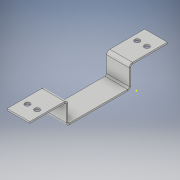
# Autodesk Inventor part: Hew battery holder
Saved by Autodesk Inventor 2017 (Build 210142000, 142)
## iProperties
Created: 2016-10-03
Part Number: Hew battery holder
Material: Generic
Document SubType Name: Sheet Metal
Designer: situh
Density: 1 g/cm^3
Sheet Metal Rule: Default
Appearance: Default
Author: situh
Autodesk Inventor part; units mm, degrees
ref_plane "YZ Plane" through (0, 0, 0) normal (1, 0, 0) x (0, 1, 0)
ref_plane "XZ Plane" through (0, 0, 0) normal (0, 1, 0) x (-1, 0, 0)
ref_plane "XY Plane" through (0, 0, 0) normal (0, 0, 1) x (1, 0, 0)
sketch "Sketch1" plane through (0, 0, 0) normal (0, 0, 1) x (1, 0, 0)
  line L0 (-22.189, 41.743) -> (-4.409, 41.743)
  line L1 (-4.409, 41.743) -> (-4.409, 23.963)
  line L2 (-4.409, 23.963) -> (-22.189, 23.963)
  line L3 (-22.189, 23.963) -> (-22.189, 41.743)
  point P0 (0, 0)
  dimension "d0" = 17.78
  dimension "d1" = 17.78
  measures "d0" distance of L2.end L0.start
  measures "d1" distance of L0.start L0.end
extrude "Plate1" add sketch "Sketch1" along normal blind 1.27
sketch "Sketch2" plane through (-4.409, 40.473, 1.27) normal (0, 1, 0) x (-1, 0, 0)
  line L0 (17.78, 0) -> (0, 0)
  line L1 (0, 0) -> (0, -30)
  line L2 (0, -30) -> (17.78, -30)
  line L3 (17.78, -30) -> (17.78, 0)
  constraints: 6 end point, 1 horizontal, 1 perpendicular, 1 vertical
edge flange "Flange1" height 30 angle 90 thickness 1.27 bend radius 1.27 thickness toward (0, 1, 0) relief straight relief width 1.27 relief depth 0.635 edges at (-13.299, 41.743, 0) wall of the first edge with corners at (-22.189, 40.473, 1.27) (-4.409, 40.473, 1.27) (-4.409, 40.473, -28.73) (-22.189, 40.473, -28.73)
bend "Bend1"
corner "Corner1"
sketch "Sketch4" plane through (-22.189, 41.743, -28.73) normal (0, 1, 0) x (1, 0, 0)
  circle A0 centre (12.7, -10.95) radius 2
  circle A1 centre (5.08, -10.95) radius 2
  line L0 (17.78, 0) -> (17.78, -27.46) projected
  line L1 (0, -27.46) -> (0, 0) projected
  line L2 (0, -27.46) -> (17.78, -27.46) projected
  point P0 (22.189, -28.73)
  dimension "d26" = 4
  dimension "d27" = 4
  dimension "d29" = 5.08
  dimension "d30" = 5.08
  dimension "d31" = 16.51
  dimension "d32" = 16.51
  constraints: 2 centre point
  measures "d26" diameter of A1
  measures "d27" diameter of A0
  measures "d29" distance from line of A0.centre L0
  measures "d30" distance from line of L1 A1.centre
  measures "d31" distance from line of L2 A1.centre
  measures "d32" vertical distance of L0.end A0.centre
extrude "Extrusion2" cut sketch "Sketch4" against normal blind 2.54
sketch "Sketch5" plane through (-4.409, 25.233, 0) normal (0, -1, 0) x (1, 0, 0)
  line L0 (-17.78, 0) -> (0, 0)
  line L1 (0, 0) -> (0, 50.8)
  line L2 (0, 50.8) -> (-17.78, 50.8)
  line L3 (-17.78, 50.8) -> (-17.78, 0)
  constraints: 6 end point, 1 horizontal, 1 perpendicular, 1 vertical
edge flange "Flange2" height 50.8 angle 90 thickness 1.27 bend radius 1.27 thickness toward (0, -1, 0) relief straight relief width 1.27 relief depth 0.635 edges at (-13.299, 23.963, 1.27) wall of the first edge with corners at (-22.189, 25.233, 0) (-4.409, 25.233, 0) (-4.409, 25.233, 50.8) (-22.189, 25.233, 50.8)
bend "Bend2"
corner "Corner2"
sketch "Sketch6" plane through (-4.409, 23.963, 49.53) normal (0, 0, 1) x (1, 0, 0)
  line L0 (-17.78, 0) -> (0, 0)
  line L1 (0, 0) -> (0, 15.24)
  line L2 (0, 15.24) -> (-17.78, 15.24)
  line L3 (-17.78, 15.24) -> (-17.78, 0)
  constraints: 6 end point, 1 horizontal, 1 perpendicular, 1 vertical
edge flange "Flange3" height 15.24 angle 90 thickness 1.27 bend radius 1.27 thickness toward (0, 0, 1) relief straight relief width 1.27 relief depth 0.635 edges at (-13.299, 25.233, 50.8) wall of the first edge with corners at (-22.189, 23.963, 49.53) (-4.409, 23.963, 49.53) (-4.409, 39.203, 49.53) (-22.189, 39.203, 49.53)
bend "Bend3"
corner "Corner3"
sketch "Sketch7" plane through (-22.189, 40.473, 52.07) normal (0, 1, 0) x (-1, 0, 0)
  line L0 (-17.78, 0) -> (0, 0)
  line L1 (0, 0) -> (0, 27.46)
  line L2 (0, 27.46) -> (-17.78, 27.46)
  line L3 (-17.78, 27.46) -> (-17.78, 0)
  constraints: 6 end point, 1 horizontal, 1 perpendicular, 1 vertical
edge flange "Flange4" height 30 angle 90 thickness 1.27 bend radius 1.27 thickness toward (0, 1, 0) relief straight relief width 1.27 relief depth 0.635 edges at (-13.299, 39.203, 50.8) wall of the first edge with corners at (-4.409, 40.473, 52.07) (-22.189, 40.473, 52.07) (-22.189, 40.473, 79.53) (-4.409, 40.473, 79.53)
bend "Bend4"
corner "Corner4"
sketch "Sketch9" plane through (-22.189, 41.743, 79.53) normal (0, 1, 0) x (1, 0, 0)
  circle A0 centre (5.08, 10.95) radius 1.9939
  circle A1 centre (12.7, 10.95) radius 1.9939
  line L0 (0, 0) -> (0, 27.46) projected
  line L1 (17.78, 27.46) -> (17.78, 0) projected
  point P0 (22.189, 79.53)
  dimension "d69" = 3.9878
  dimension "d70" = 3.9878
  dimension "d71" = 5.08
  dimension "d73" = 16.51
  dimension "d74" = 16.51
  dimension "d79" = 7.62
  constraints: 2 centre point
  measures "d69" diameter of A1
  measures "d70" diameter of A0
  measures "d71" distance from line of L0 A0.centre
  measures "d73" vertical distance of L1.start A1.centre
  measures "d74" vertical distance of L0.end A0.centre
  measures "d79" distance of A1.centre A0.centre
extrude "Extrusion4" cut sketch "Sketch9" against normal blind 5.08
sketch "Sketch10" plane through (-22.189, 25.233, 2.54) normal (0, 1, 0) x (1, 0, 0)
  point P0 (22.189, 2.54)
equation "\"d3\" = BendReliefWidth"
equation "\"d4\" = BendReliefDepth"
equation "\"d5\" = MinimumRemnant"
equation "\"d6\" = BendRadius"
equation "\"d9\" = BendRadius"
equation "\"d10\" = CornerReliefSize"
equation "\"d11\" = GapSize"
equation "\"d12\" = JacobiRadiusSize"
equation "\"d35\" = BendReliefWidth"
equation "\"d36\" = BendReliefDepth"
equation "\"d37\" = MinimumRemnant"
equation "\"d38\" = BendRadius"
equation "\"d41\" = BendRadius"
equation "\"d42\" = CornerReliefSize"
equation "\"d43\" = GapSize"
equation "\"d44\" = JacobiRadiusSize"
equation "\"d45\" = BendReliefWidth"
equation "\"d46\" = BendReliefDepth"
equation "\"d47\" = MinimumRemnant"
equation "\"d48\" = BendRadius"
equation "\"d51\" = BendRadius"
equation "\"d52\" = CornerReliefSize"
equation "\"d53\" = GapSize"
equation "\"d54\" = JacobiRadiusSize"
equation "\"d55\" = BendReliefWidth"
equation "\"d56\" = BendReliefDepth"
equation "\"d57\" = MinimumRemnant"
equation "\"d58\" = BendRadius"
equation "\"d61\" = BendRadius"
equation "\"d62\" = CornerReliefSize"
equation "\"d63\" = GapSize"
equation "\"d64\" = JacobiRadiusSize"
equation "\"BendRadius\" = Thickness"
equation "\"BendReliefWidth\" = Thickness"
equation "\"BendReliefDepth\" = 0.5 * Thickness"
equation "\"CornerReliefSize\" = 4 * Thickness"
equation "\"MinimumRemnant\" = 2 * Thickness"
equation "\"TransitionRadius\" = BendRadius"
equation "\"JacobiRadiusSize\" = Thickness"
equation "\"GapSize\" = Thickness"
equation "\"d2\" = BendRadius"
equation "\"Thickness\" = 1.27"
body "Solid1"
